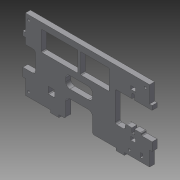
# Autodesk Inventor part: Electronics Chassis Main 6mm
Saved by Autodesk Inventor 2015 (Build 190159000, 159)
## iProperties
Created: 2014-08-06
Part Number: Electronics Chassis Main 6mm
Material: Generic
Document SubType Name: Modeling
Designer: STACKPOLE
Density: 1 g/cm^3
Appearance: Default
ChassisLength: 148.000 mm
L2: 20.000 mm
L1: 12.500 mm
Small: 5.000 mm
Large: 10.000 mm
ServoMount: 48.500 mm
Author: STACKPOLE
Autodesk Inventor part; units mm, degrees
ref_plane "YZ Plane" through (0, 0, 0) normal (1, 0, 0) x (0, 1, 0)
ref_plane "XZ Plane" through (0, 0, 0) normal (0, 1, 0) x (-1, 0, 0)
ref_plane "XY Plane" through (0, 0, 0) normal (0, 0, 1) x (1, 0, 0)
sketch "Sketch1" plane through (0, 0, 0) normal (0, 1, 0) x (-1, 0, 0)
  line L0 (148, 85) -> (0, 85)
  line L1 (0, 65) -> (-3, 65)
  line L2 (-3, 65) -> (-3, 60)
  line L3 (-3, 60) -> (0, 60)
  line L4 (0, 40) -> (148, 40) construction
  line L5 (0, 27.5) -> (-3, 27.5)
  line L6 (-3, 27.5) -> (-3, 17.5)
  line L7 (-3, 17.5) -> (0, 17.5)
  line L8 (148, 65) -> (151, 65)
  line L9 (151, 65) -> (151, 60)
  line L10 (151, 60) -> (148, 60)
  line L11 (148, 27.5) -> (151, 27.5)
  line L12 (151, 27.5) -> (151, 17.5)
  line L13 (151, 17.5) -> (148, 17.5)
  line L14 (148, 65) -> (148, 85)
  line L15 (148, 0) -> (148, 17.5)
  line L16 (148, 27.5) -> (148, 60)
  line L17 (0, 85) -> (0, 65)
  line L18 (0, 60) -> (0, 27.5)
  line L19 (0, 17.5) -> (0, 0)
  line L20 (40, 0) -> (40, -3)
  line L21 (40, -3) -> (30, -3)
  line L22 (30, -3) -> (30, 0)
  line L23 (118, 0) -> (118, -3)
  line L24 (118, -3) -> (108, -3)
  line L25 (108, -3) -> (108, 0)
  line L26 (0, 0) -> (30, 0)
  line L27 (40, 0) -> (108, 0)
  line L28 (118, 0) -> (148, 0)
  dimension "d0" = 85
  dimension "ChassisLength" = 148
  dimension "L2" = 20
  dimension "d6" = 3
  dimension "L1" = 12.5
  dimension "L3" = 20
  dimension "d41" = 10
  dimension "d42" = 3
  dimension "d44" = 30
  dimension "Small" = 5
  dimension "Large" = 10
  constraints: 58 end point, 18 parallel, 13 perpendicular, 9 horizontal, 6 collinear, 4 equal length, 4 vertical alignment, 2 horizontal alignment, 2 point on line, 1 vertical
  measures "d0" distance of L0.end L19.end
  measures "ChassisLength" distance of L19.end L15.start
  measures "L2" distance between parallel lines of L4 L3
  measures "d6" distance of L6.end L7.end
  measures "L1" distance between parallel lines of L4 L5
  measures "L3" distance between parallel lines of L0 L1
  measures "d41" distance of L23.end L24.end
  measures "d42" distance of L24.end L25.end
  measures "d44" distance between parallel lines of L19 L22
  measures "Small" distance of L1.end L2.end
  measures "Large" distance of L5.end L6.end
extrude "Extrusion1" add sketch "Sketch1" along normal blind 6
sketch "Sketch3" plane through (0, 6, 0) normal (0, 1, 0) x (1, 0, 0)
  line L0 (-148, -85) -> (0, -85) projected
  line L1 (0, 0) -> (-148, 0) projected
  line L2 (-73, -47) -> (-95, -47)
  arc A0 (-73, -47) -> (-68, -42) centre (-73, -42) ccw
  arc A1 (-100, -42) -> (-95, -47) centre (-95, -42) ccw
  line L3 (0, -17.5) -> (0, 0) projected
  line L4 (-108, 0) -> (-108, 3) projected
  line L5 (-68, 0) -> (-100, 0)
  line L6 (-95, -33) -> (-73, -33)
  line L7 (-95, -23) -> (-73, -23)
  line L8 (-100, -42) -> (-100, -38)
  line L9 (-100, -18) -> (-100, 0)
  line L10 (-68, 0) -> (-68, -18)
  line L11 (-68, -38) -> (-68, -42)
  arc A2 (-95, -33) -> (-100, -38) centre (-95, -38) ccw
  arc A3 (-68, -38) -> (-73, -33) centre (-73, -38) ccw
  arc A4 (-100, -18) -> (-95, -23) centre (-95, -18) ccw
  arc A5 (-73, -23) -> (-68, -18) centre (-73, -18) ccw
  line L12 (-148, 0) -> (-148, -17.5) projected
  point P0 (0, -6)
  point P1 (-123, 0)
  dimension "d34" = 38
  dimension "d131" = 5
  dimension "d144" = 33
  dimension "d145" = 10
  dimension "d146" = 5
  dimension "d147" = 5
  dimension "d149" = 32
  dimension "d150" = 5
  dimension "d173" = 48
  constraints: 16 end point, 14 tangent, 12 point on circle, 6 centre point, 6 perpendicular, 4 parallel, 4 point on line, 2 equal radius, 1 horizontal
  measures "d34" distance between parallel lines of L0 L2
  measures "d131" radius of A0
  measures "d144" distance between parallel lines of L1 L6
  measures "d145" distance between parallel lines of L6 L7
  measures "d146" radius of A2
  measures "d147" radius of A3
  measures "d149" distance between parallel lines of L10 L9
  measures "d150" radius of A4
  measures "d173" distance between parallel lines of L12 L9
sketch "Sketch10" plane through (0, 6, 0) normal (0, 1, 0) x (1, 0, 0)
  line L0 (0.0037, -40) -> (-151, -40) construction
  line L1 (0, -27.5) -> (3, -27.5) projected
  line L2 (0, -27.5) -> (0, -60)
  line L3 (0, -60) -> (0, -27.5) projected
  line L4 (0, -60) -> (-18, -60)
  line L5 (-18, -60) -> (-18, -66)
  line L6 (-18, -66) -> (-21, -66)
  line L7 (-21, -66) -> (-21, -60)
  line L8 (-21, -60) -> (-41, -60)
  line L9 (-41, -60) -> (-41, -24)
  line L10 (-41, -24) -> (-29, -24)
  line L11 (-29, -24) -> (-29, -30)
  line L12 (-29, -30) -> (-21, -30)
  line L13 (-21, -30) -> (-21, -24)
  line L14 (-21, -24) -> (-18, -24)
  line L15 (-18, -24) -> (-18, -30)
  line L16 (0, -27.5) -> (-10, -27.5)
  line L17 (-10, -27.5) -> (-10, -30)
  line L18 (-18, -30) -> (-10, -30)
  line L19 (-22.4, -16.5) -> (-16.6, -16.5)
  line L20 (-16.6, -16.5) -> (-16.6, -20.5)
  line L21 (-16.6, -20.5) -> (-22.4, -20.5)
  line L22 (-22.4, -20.5) -> (-22.4, -16.5)
  line L23 (-22.4, -69) -> (-16.6, -69)
  line L24 (-16.6, -69) -> (-16.6, -73)
  line L25 (-16.6, -73) -> (-22.4, -73)
  line L26 (-22.4, -73) -> (-22.4, -69)
  line L27 (-148, -27.5) -> (-136, -27.5)
  line L28 (-136, -27.5) -> (-136, -52.5)
  line L29 (-136, -52.5) -> (-148, -52.5)
  line L30 (-148, -52.5) -> (-148, -27.5)
  line L31 (-148, -60) -> (-151, -60) projected
  point P0 (0, 0)
  point P1 (-151, -27.5)
  point P2 (-19.5, -20.5)
  point P3 (-19.5, -24)
  point P4 (-136, -40)
  dimension "d158" = 12.5
  dimension "d159" = 41
  dimension "d160" = 18
  dimension "d161" = 6
  dimension "d162" = 3
  dimension "d163" = 10
  dimension "d164" = 10
  dimension "d165" = 8
  dimension "d167" = 5.8
  dimension "d168" = 4
  dimension "ServoMount" = 48.5
  dimension "d170" = 3.5
  dimension "d182" = 12
  dimension "d184" = 20
  constraints: 59 end point, 10 perpendicular, 8 horizontal, 7 parallel, 6 point on line, 4 collinear, 3 equal length, 3 midpoint, 2 vertical alignment, 1 vertical
  measures "d158" distance between parallel lines of L1 L0
  measures "d159" distance between parallel lines of L9 L2
  measures "d160" distance of L2.end L4.end
  measures "d161" distance of L4.end L5.end
  measures "d162" distance of L5.end L6.end
  measures "d163" distance of L1.start L16.end
  measures "d164" distance between parallel lines of L0 L18
  measures "d165" distance between parallel lines of L13 L11
  measures "d167" distance of L19.start L19.end
  measures "d168" distance of L19.end L20.end
  measures "ServoMount" distance between parallel lines of L23 L21
  measures "d170" distance from line of L13.end L21
  measures "d182" distance of L27.start L27.end
  measures "d184" distance of L7.end L8.end
extrude "Extrusion10" cut sketch "Sketch10" against normal through all
sketch "Sketch7" plane through (0, 0, 0) normal (0, -1, 0) x (1, 0, 0)
  line L0 (0, 85) -> (-148, 85) projected
  circle A0 centre (-144, 79.5) radius 1.5
  circle A1 centre (-144, 5.5) radius 1.5
  circle A2 centre (-5, 79.5) radius 1.5
  circle A3 centre (-24, 5.5) radius 1.5
  line L1 (0, 85) -> (0, 65) projected
  dimension "d84" = 3
  dimension "d88" = 3
  dimension "d89" = 74
  dimension "d90" = 3
  dimension "d91" = 139
  dimension "d92" = 3
  dimension "d93" = 19
  dimension "d133" = 5
  dimension "d134" = 5.5
  constraints: 4 centre point, 2 horizontal alignment, 1 vertical alignment
  measures "d84" diameter of A0
  measures "d88" diameter of A1
  measures "d89" distance between centres of A0 A1
  measures "d90" diameter of A2
  measures "d91" distance of A0.centre A2.centre
  measures "d92" diameter of A3
  measures "d93" horizontal distance of A3.centre A2.centre
  measures "d133" distance from line of L1 A2.centre
  measures "d134" distance from line of L0 A2.centre
extrude "Extrusion6" cut sketch "Sketch7" against normal through all
extrude "Extrusion8" cut sketch "Sketch3" against normal through all
fillet "Fillet10" radius 2 2 edges at (-68, 3, 0) (-100, 3, 0)
fillet "Fillet11" radius 2 4 edges at (-41, 3, 60) (-41, 3, 24) (-29, 3, 24) (-29, 3, 30)
fillet "Fillet12" radius 1 6 edges at (-21, 3, 24) (-21, 3, 66) (-18, 3, 66) (-18, 3, 24) (-10, 3, 30) (-10, 3, 27.5)
sketch "Sketch11" plane through (0, 6, 0) normal (0, 1, 0) x (1, 0, 0)
  line L0 (-121, -15) -> (-113, -15)
  line L1 (-113, -15) -> (-113, -23)
  line L2 (-113, -23) -> (-121, -23)
  line L3 (-121, -23) -> (-121, -15)
  line L4 (-73, -23) -> (-95, -23) projected
  line L5 (-118, 3) -> (-118, 0) projected
  point P0 (0, 0)
  dimension "d176" = 8
  dimension "d177" = 8
  dimension "d178" = 5
  constraints: 8 end point, 2 parallel, 1 collinear, 1 horizontal, 1 perpendicular
  measures "d176" distance of L0.end L1.end
  measures "d177" distance of L0.start L0.end
  measures "d178" distance between parallel lines of L1 L5
extrude "Extrusion11" cut sketch "Sketch11" against normal through all
fillet "Fillet13" radius 1 4 edges at (-121, 3, 15) (-113, 3, 15) (-113, 3, 23) (-121, 3, 23)
fillet "Fillet14" radius 3 2 edges at (-136, 3, 27.5) (-136, 3, 52.5)
sketch "Sketch12" plane through (0, 0, 0) normal (0, -1, 0) x (1, 0, 0)
  line L0 (-148, 85) -> (0, 85) projected
  line L1 (-41, 58) -> (-41, 26) projected
  line L2 (-136, 49.5) -> (-136, 30.5) projected
  line L3 (-11, 4.5) -> (-8, 4.5)
  line L4 (-8, 4.5) -> (-8, 9.5)
  line L5 (-8, 9.5) -> (-11, 9.5)
  line L6 (-11, 9.5) -> (-11, 4.5)
  circle A0 centre (-5, 79.5) radius 1.5 projected
  circle A1 centre (-24, 5.5) radius 1.5 projected
  line L7 (-66, 0) -> (-40, 0) projected
  point P0 (0, 0)
  dimension "d190" = 3
  dimension "d191" = 5
  dimension "d192" = 3
  dimension "d269" = 1
  constraints: 8 end point, 2 parallel, 1 horizontal, 1 perpendicular
  measures "d190" distance of L4.end L5.end
  measures "d191" distance of L3.end L4.end
  measures "d192" distance from line of A0.centre L4
  measures "d269" distance from line of A1.centre L3
extrude "Extrusion12" cut sketch "Sketch12" against normal through all
sketch "Sketch13" plane through (0, 6, 0) normal (0, 1, 0) x (1, 0, 0)
  line L0 (-48, -54) -> (-48, -78)
  line L1 (-129, -78) -> (-129, -54)
  line L2 (-41, -26) -> (-41, -58) projected
  line L3 (-136, -30.5) -> (-136, -49.5) projected
  line L4 (-73, -47) -> (-95, -47) projected
  line L5 (-148, -85) -> (0, -85) projected
  line L6 (-129, -54) -> (-85.5, -54)
  line L7 (-84, -54) -> (-84, -78) construction
  line L8 (-85.5, -54) -> (-85.5, -78)
  line L9 (-82.5, -54) -> (-82.5, -78)
  line L10 (-82.5, -54) -> (-48, -54)
  line L11 (-85.5, -78) -> (-129, -78)
  line L12 (-82.5, -78) -> (-48, -78)
  line L13 (-85.5, -54) -> (-82.5, -54) construction
  point P0 (0, 0)
  point P1 (-84, -47)
  dimension "d201" = 7
  dimension "d203" = 7
  dimension "d266" = 7
  dimension "d267" = 7
  dimension "d268" = 3
  constraints: 20 end point, 4 horizontal, 4 perpendicular, 3 parallel, 2 midpoint, 1 collinear, 1 vertical, 1 vertical alignment
  measures "d201" distance between parallel lines of L2 L0
  measures "d203" distance between parallel lines of L3 L1
  measures "d266" distance between parallel lines of L4 L6
  measures "d267" distance between parallel lines of L5 L11
  measures "d268" distance of L6.end L9.start
extrude "Extrusion13" cut sketch "Sketch13" against normal through all
fillet "Fillet16" radius 1 8 edges at (-48, 3, 54) (-48, 3, 78) (-129, 3, 54) (-129, 3, 78) (-82.5, 3, 54) (-82.5, 3, 78) (-85.5, 3, 78) (-85.5, 3, 54)
body "Solid1"
